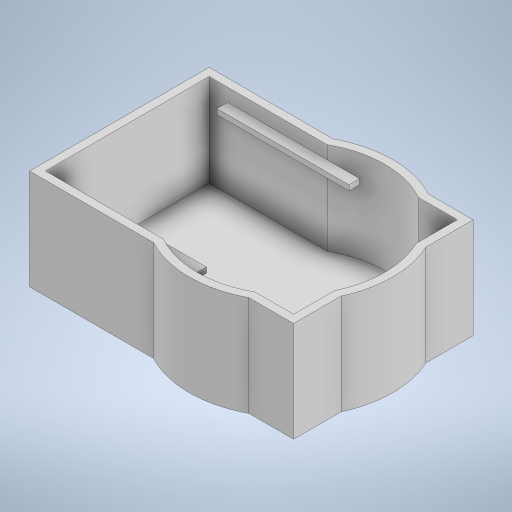
# Autodesk Inventor part: Box Base Plate
Saved by Autodesk Inventor 2023 (Build 270158000, 158)
## iProperties
Created: 2022-10-24
Part Number: Box Base Plate
Material: Generic
Document SubType Name: Modeling
Designer: cheng
Density: 1 g/cm^3
Appearance: Default
Author: cheng
Autodesk Inventor part; units mm, degrees
ref_plane "YZ Plane" through (0, 0, 0) normal (1, 0, 0) x (0, 1, 0)
ref_plane "XZ Plane" through (0, 0, 0) normal (0, 1, 0) x (-1, 0, 0)
ref_plane "XY Plane" through (0, 0, 0) normal (0, 0, 1) x (1, 0, 0)
sketch "Sketch1" plane through (0, 0, 0) normal (0, 1, 0) x (-1, 0, 0)
  line L0 (500, -340) -> (-500, -340)
  line L1 (-500, -340) -> (-500, 340)
  line L2 (-500, 340) -> (500, 340)
  line L3 (500, 340) -> (500, -340)
  line L4 (500, -340) -> (-500, 340) construction
  line L5 (-500, -340) -> (500, 340) construction
  circle A0 centre (-150, 0) radius 335
  circle A1 centre (-150, 0) radius 385
  point P0 (0, 0)
  point P1 (-500, 0)
  point P2 (-495, 0)
  point P3 (-495, -64.0312)
  point P4 (30.6239, 340)
  point P5 (-330.6239, 340)
  point P6 (-500, 160.3901)
  point P7 (-500, -160.3901)
  point P8 (-330.6239, -340)
  point P9 (30.6239, -340)
  dimension "d0" = 1000
  dimension "d1" = 680
  dimension "d2" = 670
  dimension "d3" = 350
  dimension "d6" = 50
  constraints: 12 end point, 3 midpoint, 2 centre point, 2 parallel, 1 coincident, 1 horizontal, 1 perpendicular
  measures "d0" distance of L0.start L0.end
  measures "d1" distance of L0.end L1.end
  measures "d2" diameter of A0
  measures "d3" distance of point (-500, 0) A0.centre
  measures "d6" radial gap between concentric circles of A0 A1
extrude "Extrusion1" add sketch "Sketch1" along normal blind 30 contours L0 A1 L2 L3 | A1 L0 | L0 A1 L1 L2 | L0 L1 A1 | L2 A1 | A1 L1 | A1 L1 L2 | A0
sketch "Sketch3" plane through (0, 30, 0) normal (0, 1, 0) x (1, 0, 0)
  arc A0 (330.6239, 340) -> (-30.6239, 340) centre (150, 0) ccw projected
  line L0 (330.6239, -340) -> (500, -340) projected
  line L1 (-30.6239, 340) -> (330.6239, -340)
  line L2 (500, 340) -> (330.6239, 340) projected
  line L3 (330.6239, 340) -> (-30.6239, -340)
  circle A1 centre (150, 0) radius 385
  circle A2 centre (150, 0) radius 355
  line L4 (-30.6239, 340) -> (-500, 340) projected
  line L5 (-500, 340) -> (-500, -340) projected
  line L6 (-500, -340) -> (-30.6239, -340) projected
  line L7 (500, -340) -> (500, -160.3901) projected
  line L8 (500, 160.3901) -> (500, 340) projected
  arc A3 (330.6239, 340) -> (-30.6239, 340) centre (150, 0) ccw projected
  arc A4 (-30.6239, -340) -> (330.6239, -340) centre (150, 0) ccw projected
  line L9 (470, 310) -> (-470, 310)
  line L10 (-470, 310) -> (-470, -310)
  line L11 (-470, -310) -> (470, -310)
  line L12 (470, -310) -> (470, 310)
  line L13 (470, 310) -> (-470, -310) construction
  line L14 (-470, 310) -> (470, -310) construction
  point P0 (0, 0)
  point P1 (-30.6239, -340)
  point P2 (-22.9884, -310)
  point P3 (-22.9884, 310)
  point P4 (322.9884, 310)
  point P5 (470, 153.7043)
  point P6 (470, -153.7043)
  point P7 (322.9884, -310)
  dimension "d7" = 30
  dimension "d8" = 30
  dimension "d9" = 30
  constraints: 16 end point, 2 centre point, 2 coincident, 2 midpoint, 2 parallel, 1 horizontal, 1 perpendicular
  measures "d7" distance between parallel lines of L4 L9
  measures "d8" distance between parallel lines of L5 L10
  measures "d9" radial gap between concentric circles of A0 A2
extrude "Extrusion2" add sketch "Sketch3" along normal blind 350 contours L3 A2 L1 A0 | A1 L9 A2 L3 | L2 L8 A1 L12 L9 | L1 A2 L9 A1 | A1 L9 L10 L11 L6 L5 L4 | A1 L12 A2 | L11 A2 L3 A1 | L3 A2 L1 A1 | L7 L0 A1 L11 L12 | L1 A2 L11 A1
sketch "Sketch4" plane through (-470, 30, -310) normal (0, 0, 1) x (1, 0, 0)
  line L0 (70, 300) -> (570, 300)
  line L1 (570, 300) -> (570, 280)
  line L2 (570, 280) -> (70, 280)
  line L3 (70, 280) -> (70, 300)
  line L4 (0, 0) -> (0, 350) projected
  line L5 (0, 350) -> (447.0116, 350) projected
  point P0 (470, -30)
  point P1 (570, 290)
  dimension "d12" = 70
  dimension "d13" = 500
  dimension "d14" = 20
  dimension "d15" = 50
  constraints: 8 end point, 2 parallel, 1 horizontal, 1 midpoint, 1 perpendicular
  measures "d12" distance between parallel lines of L4 L3
  measures "d13" distance from line of point (570, 290) L3
  measures "d14" distance between parallel lines of L2 L0
  measures "d15" distance between parallel lines of L5 L0
extrude "Extrusion3" add sketch "Sketch4" along normal blind 40
sketch "Sketch5" plane through (-22.9884, 30, 310) normal (0, 0, -1) x (-1, 0, 0)
  line L0 (377.0116, 300) -> (-122.9884, 300)
  line L1 (-122.9884, 300) -> (-122.9884, 280)
  line L2 (-122.9884, 280) -> (377.0116, 280)
  line L3 (377.0116, 280) -> (377.0116, 300)
  line L4 (0, 350) -> (447.0116, 350) projected
  line L5 (447.0116, 0) -> (447.0116, 350) projected
  point P0 (-22.9884, -30)
  dimension "d18" = 50
  dimension "d19" = 20
  dimension "d20" = 70
  dimension "d21" = 500
  constraints: 8 end point, 2 parallel, 1 horizontal, 1 perpendicular
  measures "d18" distance between parallel lines of L4 L0
  measures "d19" distance between parallel lines of L2 L0
  measures "d20" distance between parallel lines of L5 L3
  measures "d21" distance between parallel lines of L3 L1
extrude "Extrusion4" add sketch "Sketch5" along normal blind 40
body "Solid1"
